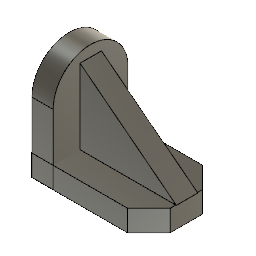
A1 (Autodesk Fusion 360 design; units mm, degrees)
Autodesk Fusion 360 part; units mm, degrees
sketch "Sketch1" plane through (0, 0, 0) normal (0, 0, 1) x (1, 0, 0)
  line L0 (33, -21) -> (-33, -21)
  line L1 (-33, -21) -> (-33, 21)
  line L2 (-33, 21) -> (33, 21)
  line L3 (33, 21) -> (33, -21)
  line L4 (33, -21) -> (-33, 21) construction
  line L5 (-33, -21) -> (33, 21) construction
  dimension "d1" = 66
  dimension "d2" = 42
  constraint horizontal L0
  constraint perpendicular L0 L1
  constraint parallel L0 L2
  constraint parallel L1 L3
  constraint coincident L4 origin
  constraint coincident L5 origin
  measures "d1" distance of L1.end L2.end
  measures "d2" distance of L0.end L1.end
extrude "Extrude1" add sketch "Sketch1" along normal blind 12 makes body 1
chamfer "Chamfer1" distance 12 angle 45 2 edges at (33, -21, 6) (33, 21, 6) on bodies 1
sketch "Sketch2" plane through (0, 0, 0) normal (0, 0, 1) x (1, 0, 0)
  line L0 (-32.7988, 21.1552) -> (-20.7988, 21.1552)
  line L1 (-20.7988, 21.1552) -> (-20.7988, -20.8448)
  line L2 (-20.7988, -20.8448) -> (-32.7988, -20.8448)
  line L3 (-32.7988, -20.8448) -> (-32.7988, 21.1552)
  dimension "d6" = 12
  dimension "d7" = 42
  constraint horizontal L0
  constraint vertical L1
  constraint horizontal L2
  constraint vertical L3
  measures "d6" distance of L0.start L0.end
  measures "d7" distance of L0.start L2.end
extrude "Extrude2" add sketch "Sketch2" along normal blind 60 separate body makes body 2
fillet "Fillet1" radius 21 2 edges at (-26.7988, -20.8448, 60) (-26.7988, 21.1552, 60) on bodies 2
sketch "Sketch3" plane through (0, 0, 0) normal (0, 1, 0) x (1, 0, 0)
  line L0 (-20.5897, -54.0952) -> (-20.5897, -12.0952)
  line L1 (-20.5897, -12.0952) -> (33.4103, -12.0952)
  line L2 (33.4103, -12.0952) -> (-20.5897, -54.0952)
  dimension "d11" = 42
  dimension "d12" = 54
  constraint vertical L0
  constraint perpendicular L0 L1
  measures "d11" distance of L0.start L0.end
  measures "d12" distance of L0.end L1.end
extrude "Extrude3" add sketch "Sketch3" along normal mid plane 12 separate body makes body 3
